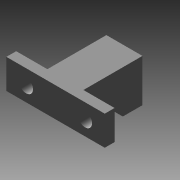
# Autodesk Inventor part: Platform Adapter
Saved by Autodesk Inventor 2015 (Build 190159000, 159)
## iProperties
Created: 2015-04-23
Part Number: Platform Adapter
Material: Generic
Document SubType Name: Modeling
Designer: pltwe4
Density: 1 g/cm^3
Appearance: Default
Author: pltwe4
Autodesk Inventor part; units mm, degrees
ref_plane "YZ Plane" through (0, 0, 0) normal (1, 0, 0) x (0, 1, 0)
ref_plane "XZ Plane" through (0, 0, 0) normal (0, 1, 0) x (-1, 0, 0)
ref_plane "XY Plane" through (0, 0, 0) normal (0, 0, 1) x (1, 0, 0)
sketch "Sketch1" plane through (0, 0, 0) normal (0, 1, 0) x (-1, 0, 0)
  line L0 (-15, 4.5) -> (15, 4.5)
  line L1 (15, 4.5) -> (15, -4.5)
  line L2 (15, -4.5) -> (-15, -4.5)
  line L3 (-15, -4.5) -> (-15, 4.5)
  line L4 (-15, 4.5) -> (15, -4.5) construction
  line L5 (15, 4.5) -> (-15, -4.5) construction
  circle A0 centre (9, 0) radius 2.125
  circle A1 centre (-9, 0) radius 2.125
  line L6 (0, -6.3) -> (0, 6.3) projected
  line L7 (-21, 0) -> (21, 0) projected
  point P0 (0, 0)
  dimension "d0" = 9
  dimension "d1" = 30
  dimension "d2" = 4.25
  dimension "d4" = 18
  constraints: 12 end point, 2 centre point, 2 midpoint, 2 parallel, 1 equal radius, 1 horizontal, 1 perpendicular, 1 point on line, 1 other
  measures "d0" distance of L0.end L1.end
  measures "d1" distance of L0.start L0.end
  measures "d2" diameter of A0
  measures "d4" distance of A1.centre A0.centre
extrude "Extrusion1" add sketch "Sketch1" along normal blind 3 contours L0 L6 L7 A1 L3 | L0 L1 L7 A0 L6 | L7 A1 L6 L2 L3 | L7 A0 L1 L2 L6
sketch "Sketch2" plane through (0, 3, 0) normal (0, 1, 0) x (1, 0, 0)
  circle A0 centre (9, 0) radius 2.125 projected
  circle A1 centre (-9, 0) radius 2.125 projected
  line L0 (-15, -4.5) -> (15, -4.5) projected
  line L1 (15, -4.5) -> (15, 4.5) projected
  line L2 (15, 4.5) -> (-15, 4.5) projected
  line L3 (-15, 4.5) -> (-15, -4.5) projected
  line L4 (5.5, -4.5) -> (-5.5, -4.5)
  line L5 (-5.5, -4.5) -> (-5.5, 4.5)
  line L6 (-5.5, 4.5) -> (5.5, 4.5)
  line L7 (5.5, 4.5) -> (5.5, -4.5)
  line L8 (5.5, -4.5) -> (-5.5, 4.5) construction
  line L9 (-5.5, -4.5) -> (5.5, 4.5) construction
  point P0 (0, 0)
  dimension "d7" = 11
  constraints: 12 end point, 2 midpoint, 2 parallel, 1 horizontal, 1 perpendicular, 1 point on line
  measures "d7" distance between parallel lines of L7 L5
extrude "Extrusion2" add sketch "Sketch2" along normal blind 18 contours L5 L2 L7 L0
sketch "Sketch3" plane through (0, 21, 0) normal (0, 1, 0) x (1, 0, 0)
  line L0 (-5.5, 4.5) -> (-5.5, -4.5) projected
  line L1 (-5.5, -4.5) -> (5.5, -4.5) projected
  line L2 (5.5, -4.5) -> (5.5, 4.5) projected
  line L3 (5.5, 4.5) -> (-5.5, 4.5) projected
  line L4 (-5.5, -4.5) -> (-5.5, 4.5) projected
  line L5 (-5.5, 2.5) -> (5.5, 2.5)
  point P0 (0, 0)
  dimension "d10" = 2
  constraints: 2 end point, 2 point on line, 1 perpendicular
  measures "d10" distance between parallel lines of L3 L5
extrude "Extrusion3" cut sketch "Sketch3" against normal blind 13 contours L3 L2 L5 L0
sketch "Sketch4" plane through (5.5, 21, -2.5) normal (0, 0, -1) x (-1, 0, 0)
  line L0 (0, 0) -> (11, 0) projected
  line L1 (0, -13) -> (0, 0) projected
  line L2 (0, -13) -> (11, -13) projected
  line L3 (11, 0) -> (11, -13) projected
  line L4 (0, -6) -> (11, -6)
  point P0 (5.5, -21)
  dimension "d13" = 6
  constraints: 2 end point, 2 point on line, 1 perpendicular
  measures "d13" distance between parallel lines of L0 L4
extrude "Extrusion4" add sketch "Sketch4" along normal blind 6 contours L0 L3 L4 L1
body "Solid1"
